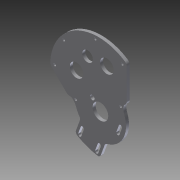
# Autodesk Inventor part: front plate
Saved by Autodesk Inventor 2012 (Build 160160000, 160)
## iProperties
Created: 2012-02-09
Part Number: front plate
Material: Default
Document SubType Name: Modeling
Designer: caduser
Density: 1 g/cm^3
Author: caduser
Autodesk Inventor part; units mm, degrees
ref_plane "YZ Plane" through (0, 0, 0) normal (1, 0, 0) x (0, 1, 0)
ref_plane "XZ Plane" through (0, 0, 0) normal (0, 1, 0) x (-1, 0, 0)
ref_plane "XY Plane" through (0, 0, 0) normal (0, 0, 1) x (1, 0, 0)
sketch "Sketch1" plane through (0, 0, 0) normal (0, 0, 1) x (1, 0, 0)
  line L0 (-176.0344, 0) -> (115.3938, 0) projected
  line L1 (0, -134.9094) -> (0, 212.5709) projected
  line L2 (0, 0) -> (-134.4018, 134.4018) construction
  circle A0 centre (0, 0) radius 16.51
  circle A1 centre (-64.8398, 5.6727) radius 6.35 construction
  circle A2 centre (46.0238, 46.0238) radius 6.35 construction
  arc A3 (-51.2387, -16.9675) -> (-59.3872, -5.1957) centre (-75.3511, -24.9522) ccw
  arc A4 (48.833, 34.1932) -> (50.1576, 19.9378) centre (73.7612, 29.3203) ccw
  circle A5 centre (0, 0) radius 53.975 construction
  circle A6 centre (-50.2894, 50.2894) radius 14.2875
  circle A7 centre (-26.9875, 87.3943) radius 11.1125
  circle A8 centre (13.589, 89.6653) radius 14.2875
  arc A9 (51.2312, 117.4993) -> (-105.7834, 37.5874) centre (-4.3145, 32.4274) ccw
  line L3 (-103.0059, 30.3685) -> (-71.575, -1.0624)
  line L4 (55.5488, 46.0238) -> (55.5488, 109.5238)
  arc A10 (55.5488, 109.5238) -> (51.2312, 117.4993) centre (46.0238, 109.5238) ccw
  arc A11 (-105.7834, 37.5874) -> (-103.0059, 30.3685) centre (-96.2707, 37.1036) ccw
  arc A12 (-71.575, -1.0624) -> (-63.9628, -3.8118) centre (-64.8398, 5.6727) ccw
  arc A13 (51.4486, 38.1945) -> (55.5488, 46.0238) centre (46.0238, 46.0238) ccw
  line L5 (0, 0) -> (-64.8398, 5.6727) construction
  arc A14 (-59.3872, -5.1957) -> (-63.9628, -3.8118) centre (-63.3782, -10.1348) ccw
  arc A15 (51.4486, 38.1945) -> (48.833, 34.1932) centre (55.0651, 32.975) ccw
  line L6 (0, 0) -> (46.0238, 46.0238) construction
  line L7 (-59.3872, -5.1957) -> (0, 0) construction
  line L8 (48.833, 34.1932) -> (0, 0) construction
  line L9 (0, 0) -> (-28.2338, -77.5716) construction
  line L10 (0.6691, -79.3887) -> (9.0934, -56.243)
  line L11 (-43.1182, -37.2395) -> (-51.5426, -60.3852)
  arc A16 (-51.2387, -16.9675) -> (-43.9184, -31.3763) centre (0, 0) ccw
  arc A17 (13.4752, -52.2659) -> (50.1576, 19.9378) centre (0, 0) ccw
  arc A18 (-48.7265, -68.0701) -> (-6.4279, -83.4655) centre (17.2205, 47.3129) ccw
  arc A19 (-43.1182, -37.2395) -> (-43.9184, -31.3763) centre (-49.0853, -35.0676) ccw
  arc A20 (-51.5426, -60.3852) -> (-48.7265, -68.0701) centre (-45.5755, -62.557) ccw
  arc A21 (-6.4279, -83.4655) -> (0.6691, -79.3887) centre (-5.298, -77.2168) ccw
  arc A22 (13.4752, -52.2659) -> (9.0934, -56.243) centre (15.0605, -58.4148) ccw
  circle A23 centre (-17.0625, 17.0625) radius 4.7625 construction
  point P0 (55.5488, 114.5184)
  point P1 (-105.911, 33.2736)
  point P2 (-1.1237, -84.3143)
  point P3 (-41.9333, -33.9838)
  point P4 (-53.3354, -65.3108)
  point P5 (10.2784, -52.9873)
  dimension "d1" = 33.02
  dimension "d5" = 12.7
  dimension "d11" = 25.4
  dimension "d14" = 45
  dimension "d16" = 107.95
  dimension "d19" = 28.575
  dimension "d22" = 22.225
  dimension "d25" = 43.815
  dimension "d27" = 28.575
  dimension "d29" = 40.64
  dimension "d30" = 9.525
  dimension "d31" = 9.525
  dimension "d34" = 63.5
  dimension "d35" = 101.6
  dimension "d36" = 44.45
  dimension "d38" = 6.35
  dimension "d39" = 6.35
  dimension "d43" = 65.0875
  dimension "d44" = 130
  dimension "d45" = 5
  dimension "d46" = 35
  dimension "d57" = 20
  dimension "d58" = 27.7812
  dimension "d60" = 33.3375
  dimension "d61" = 33.3375
  dimension "d63" = 82.55
  dimension "d64" = 6.35
  dimension "d83" = 24.13
  dimension "d84" = 9.525
  dimension "d85" = 46.99
  dimension "d86" = 26.9875
  dimension "d87" = 13.589
  constraints: 42 point on circle, 24 centre point, 20 end point, 20 tangent, 8 point on line, 7 equal radius, 6 coincident, 4 parallel, 1 equal length, 1 perpendicular
  measures "d1" diameter of A0
  measures "d5" diameter of A1
  measures "d11" radius of A3
  measures "d14" angle of L1 L2
  measures "d16" diameter of A5
  measures "d19" diameter of A6
  measures "d22" diameter of A7
  measures "d25" distance of A7.centre A6.centre
  measures "d27" diameter of A8
  measures "d29" distance of A8.centre A7.centre
  measures "d30" radius of A10
  measures "d31" radius of A12
  measures "d34" distance of L4.start L4.end
  measures "d35" radius of A9
  measures "d36" distance of L3.start L3.end
  measures "d38" radius of A14
  measures "d39" radius of A15
  measures "d43" distance of L5.start L6.end
  measures "d44" angle of L6 L5
  measures "d45" angle of L0 L7
  measures "d46" angle of L0 L8
  measures "d57" angle of L1 L9
  measures "d58" distance between parallel lines of L10 L9
  measures "d60" distance of A5.start point (-53.335, -65.311)
  measures "d61" distance of point (-1.124, -84.314) A5.end
  measures "d63" distance of L5.start L9.end
  measures "d64" radius of A19
  measures "d83" distance of A23.centre L2.start
  measures "d84" diameter of A23
  measures "d85" distance of A6.centre A23.centre
  measures "d86" distance from line of L1 A7.centre
  measures "d87" distance from line of L1 A8.centre
extrude "Base" add sketch "Sketch1" along normal mid plane 6.35 contours L3 A11 A9 L1 A8 A0 L0 | L0 A0 L1 A21 A18 A20 L11 A19 A16 A3 A14 A12 L3 | L1 A8 A9 A10 L4 A13 A15 A4 A17 L0 A0 | A0 L0 A17 A22 L10 A21 L1
sketch "Sketch2" plane through (0, 0, -3.175) normal (0, 0, -1) x (-1, 0, 0)
  arc A0 (103.0059, 30.3685) -> (105.7834, 37.5874) centre (96.2707, 37.1036) ccw projected
  arc A1 (-51.2312, 117.4993) -> (-55.5488, 109.5238) centre (-46.0238, 109.5238) ccw projected
  arc A2 (-50.1576, 19.9378) -> (-13.4752, -52.2659) centre (0, 0) ccw projected
  line L0 (141.1514, 0) -> (-101.0644, 0) projected
  line L1 (0, -127.0857) -> (0, 177.5463) projected
  line L2 (0, 0) -> (11.1042, 126.9216) construction
  line L3 (0, 0) -> (77.2258, 92.0341) construction
  dimension "d88" = 5
  dimension "d89" = 40
  dimension "d90" = 127.4064
  dimension "d91" = 120.142
  constraints: 4 end point, 2 coincident
  measures "d88" angle of L1 L2
  measures "d89" angle of L1 L3
  measures "d90" distance of L2.start L2.end
  measures "d91" distance of L2.start L3.end
hole "Standoff Holes" at (46.0238, 109.5238, -3.175) at (-96.2707, 37.1036, -3.175) at (-77.2258, 92.0341, -3.175) at (-11.1042, 126.9216, -3.175) direction (0, 0, 1) diameter 5.1054 end through all counterbore diameter 9.779 counterbore depth 1.5875 clearance for "Flat Head Machine Screw (82)" size "#10" standard "Ansi Unified Screw Threads"
sketch "Sketch4" plane through (0, 0, 3.175) normal (0, 0, 1) x (1, 0, 0)
  line L0 (9.0934, -56.243) -> (0.6691, -79.3887) projected
  arc A0 (-46.8486, -63.1399) -> (-40.4997, -65.4507) centre (-43.6742, -64.2953) ccw
  arc A1 (-11.0463, -76.1709) -> (-4.6974, -78.4817) centre (-7.8719, -77.3263) ccw
  arc A2 (-35.0701, -50.5331) -> (-41.4191, -48.2223) centre (-38.2446, -49.3777) ccw
  arc A3 (0.7322, -63.5641) -> (-5.6168, -61.2532) centre (-2.4423, -62.4087) ccw
  line L1 (-40.4997, -65.4507) -> (-35.0701, -50.5331)
  line L2 (-46.8486, -63.1399) -> (-41.4191, -48.2223)
  line L3 (-11.0463, -76.1709) -> (-5.6168, -61.2532)
  line L4 (0.7322, -63.5641) -> (-4.6974, -78.4817)
  line L5 (-7.8719, -77.3263) -> (-43.6742, -64.2953) construction
  arc A4 (-48.7265, -68.0701) -> (-6.4279, -83.4655) centre (17.2205, 47.3129) ccw projected
  arc A5 (33.6371, -20.1122) -> (39.9861, -22.423) centre (36.8116, -21.2676) ccw
  arc A6 (45.4156, -7.5054) -> (39.0667, -5.1946) centre (42.2412, -6.35) ccw
  line L6 (39.9861, -22.423) -> (45.4156, -7.5054)
  line L7 (39.0667, -5.1946) -> (33.6371, -20.1122)
  line L8 (-140.2473, 0) -> (100.9137, 0) projected
  line L9 (0, -129.1287) -> (0, 177.8868) projected
  arc A7 (13.4752, -52.2659) -> (50.1576, 19.9378) centre (0, 0) ccw projected
  dimension "d66" = 6.7564
  dimension "d70" = 15.875
  dimension "d71" = 38.1
  dimension "d72" = 5.353
  dimension "d73" = 2.3813
  dimension "d74" = 15.875
  dimension "d75" = 6.7564
  dimension "d76" = 15.875
  dimension "d77" = 6.35
  dimension "d78" = 45.2437
  constraints: 14 end point, 12 point on circle, 10 tangent, 6 centre point, 5 parallel, 4 equal radius, 1 perpendicular
  measures "d66" distance between parallel lines of L3 L4
  measures "d70" distance of L2.start L2.end
  measures "d71" distance of L5.start L5.end
  measures "d72" distance between parallel lines of L4 L0
  measures "d74" distance of L3.start L3.end
  measures "d75" distance between parallel lines of L7 L6
  measures "d76" distance of L7.start L7.end
  measures "d77" distance from line of L8 A6.centre
  measures "d78" distance from line of L6 A7.centre
extrude "Tensioning Slots" cut sketch "Sketch4" against normal through all
sketch "Sketch5" plane through (0, 0, 3.175) normal (0, 0, 1) x (1, 0, 0)
  circle A0 centre (0, 0) radius 16.51 projected
  circle A1 centre (-50.2894, 50.2894) radius 14.2875 projected
  arc A2 (13.4752, -52.2659) -> (50.1576, 19.9378) centre (0, 0) ccw projected
  line L0 (-71.575, -1.0624) -> (-103.0059, 30.3685) projected
  line L1 (0, 0) -> (-50.2894, 50.2894) construction
  circle A3 centre (-17.0625, 17.0625) radius 4.7752
  line L2 (-140.2473, 0) -> (100.9137, 0) projected
  line L3 (0, -127.0857) -> (0, 177.5463) projected
  dimension "d79" = 9.5504
  dimension "d80" = 24.13
  constraints: 2 end point, 1 centre point, 1 parallel, 1 point on line
  measures "d79" diameter of A3
  measures "d80" distance of A3.centre A0.centre
extrude "Idler Bearing Hole" cut sketch "Sketch5" against normal through all contours A3
sketch "Sketch6" plane through (0, 0, -3.175) normal (0, 0, -1) x (-1, 0, 0)
  arc A0 (63.9628, -3.8118) -> (71.575, -1.0624) centre (64.8398, 5.6727) ccw projected
  arc A1 (-55.5488, 46.0238) -> (-51.4486, 38.1945) centre (-46.0238, 46.0238) ccw projected
  line L0 (140.2473, 0) -> (-100.9137, 0) projected
  line L1 (0, -127.0857) -> (0, 177.5463) projected
  circle A2 centre (-42.5172, 30.5409) radius 6.35 construction
  circle A3 centre (52.2014, -3.9338) radius 6.35 construction
  arc A4 (-50.1576, 19.9378) -> (-13.4752, -52.2659) centre (0, 0) ccw projected
  line L2 (0, 0) -> (-42.5172, 30.5409) construction
  line L3 (0, 0) -> (52.2014, -3.9338) construction
  dimension "d92" = 12.7
  dimension "d93" = 15.875
  dimension "d94" = 15.875
  dimension "d102" = 52.3494
  dimension "d103" = 52.3494
  constraints: 4 end point, 2 centre point, 2 coincident, 1 equal radius
  measures "d92" diameter of A2
  measures "d93" distance of A1.centre point (-42.517, 30.541)
  measures "d94" distance of A0.centre point (52.201, -3.934)
  measures "d102" distance of L2.start L2.end
  measures "d103" distance of L2.start L3.end
hole "Standoff holes to motor plate" at (42.5172, 30.5409, -3.175) at (-52.2014, -3.9338, -3.175) direction (0, 0, 1) diameter 5.1054 end through all counterbore diameter 9.779 counterbore depth 1.5875 clearance for "Flat Head Machine Screw (82)" size "#10" standard "Ansi Unified Screw Threads"
body "Solid1"
